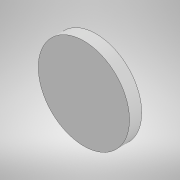
# Autodesk Inventor part: 통풍구
Saved by Autodesk Inventor 2022 (Build 260153000, 153)
## iProperties
Created: 2024-07-11
Part Number: 통풍구
Material: 일반
Document SubType Name: Modeling
Designer: seama
Density: 1 g/cm^3
Appearance: 기본값
Author: seama
Autodesk Inventor part; units mm, degrees
ref_plane "우측면도" through (0, 0, 0) normal (1, 0, 0) x (0, 1, 0)
ref_plane "평면도" through (0, 0, 0) normal (0, 1, 0) x (-1, 0, 0)
ref_plane "정면도" through (0, 0, 0) normal (0, 0, 1) x (1, 0, 0)
sketch "스케치1" plane through (0, 0, 0) normal (0, 0, 1) x (1, 0, 0)
  circle A0 centre (0, 0) radius 14.9
  dimension "d0" = 29.8
  constraints: 1 centre point, 1 coincident
  measures "d0" diameter of A0
extrude "돌출1" add sketch "스케치1" along normal blind 4
